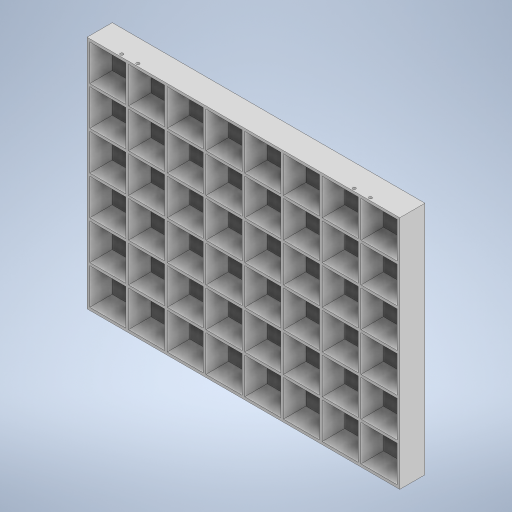
# Autodesk Inventor part: RatPelletBox_v05
Saved by Autodesk Inventor 2024 (Build 280153000, 153)
## iProperties
Created: 2025-06-19
Part Number: RatPelletBox_v05
Material: Generic
Document SubType Name: Modeling
Designer: Akramilab
Density: 1 g/cm^3
Appearance: Default
Author: Akramilab
Autodesk Inventor part; units mm, degrees
ref_plane "YZ Plane" through (0, 0, 0) normal (1, 0, 0) x (0, 1, 0)
ref_plane "XZ Plane" through (0, 0, 0) normal (0, 1, 0) x (-1, 0, 0)
ref_plane "XY Plane" through (0, 0, 0) normal (0, 0, 1) x (1, 0, 0)
sketch "Sketch1" plane through (0, 0, 0) normal (0, 0, 1) x (1, 0, 0)
  line L0 (-173.5, -130.5) -> (173.5, -130.5)
  line L1 (173.5, -130.5) -> (173.5, 130.5)
  line L2 (173.5, 130.5) -> (-173.5, 130.5)
  line L3 (-173.5, 130.5) -> (-173.5, -130.5)
  line L4 (-173.5, -130.5) -> (173.5, 130.5) construction
  line L5 (173.5, -130.5) -> (-173.5, 130.5) construction
  point P0 (0, 0)
  dimension "d0" = 347
  dimension "d1" = 261
  constraints: 12 end point, 2 midpoint, 2 parallel, 1 horizontal, 1 perpendicular
  measures "d0" distance of L1.end L2.end
  measures "d1" distance of L0.end L1.end
extrude "Extrusion1" add sketch "Sketch1" along normal blind 28
sketch "Sketch2" plane through (0, 0, 28) normal (0, 0, 1) x (1, 0, 0)
  line L0 (-170.5, 127.5) -> (-130.5, 127.5)
  line L1 (-130.5, 127.5) -> (-130.5, 87.5)
  line L2 (-130.5, 87.5) -> (-170.5, 87.5)
  line L3 (-170.5, 87.5) -> (-170.5, 127.5)
  line L4 (-170.5, 127.5) -> (-130.5, 87.5) construction
  line L5 (-130.5, 127.5) -> (-170.5, 87.5) construction
  line L6 (173.5, 130.5) -> (-173.5, 130.5) projected
  line L7 (-173.5, 130.5) -> (-173.5, -130.5) projected
  line L8 (-127.5, 127.5) -> (-87.5, 127.5)
  line L9 (-87.5, 127.5) -> (-87.5, 87.5)
  line L10 (-87.5, 87.5) -> (-127.5, 87.5)
  line L11 (-127.5, 87.5) -> (-127.5, 127.5)
  line L12 (-127.5, 127.5) -> (-87.5, 87.5) construction
  line L13 (-87.5, 127.5) -> (-127.5, 87.5) construction
  line L14 (-84.5, 127.5) -> (-44.5, 127.5)
  line L15 (-44.5, 127.5) -> (-44.5, 87.5)
  line L16 (-44.5, 87.5) -> (-84.5, 87.5)
  line L17 (-84.5, 87.5) -> (-84.5, 127.5)
  line L18 (-84.5, 127.5) -> (-44.5, 87.5) construction
  line L19 (-44.5, 127.5) -> (-84.5, 87.5) construction
  line L20 (-41.5, 127.5) -> (-1.5, 127.5)
  line L21 (-1.5, 127.5) -> (-1.5, 87.5)
  line L22 (-1.5, 87.5) -> (-41.5, 87.5)
  line L23 (-41.5, 87.5) -> (-41.5, 127.5)
  line L24 (-41.5, 127.5) -> (-1.5, 87.5) construction
  line L25 (-1.5, 127.5) -> (-41.5, 87.5) construction
  line L26 (1.5, 127.5) -> (41.5, 127.5)
  line L27 (41.5, 127.5) -> (41.5, 87.5)
  line L28 (41.5, 87.5) -> (1.5, 87.5)
  line L29 (1.5, 87.5) -> (1.5, 127.5)
  line L30 (1.5, 127.5) -> (41.5, 87.5) construction
  line L31 (41.5, 127.5) -> (1.5, 87.5) construction
  line L32 (-170.5, 84.5) -> (-130.5, 84.5)
  line L33 (-130.5, 84.5) -> (-130.5, 44.5)
  line L34 (-130.5, 44.5) -> (-170.5, 44.5)
  line L35 (-170.5, 44.5) -> (-170.5, 84.5)
  line L36 (-170.5, 84.5) -> (-130.5, 44.5) construction
  line L37 (-130.5, 84.5) -> (-170.5, 44.5) construction
  line L38 (-127.5, 84.5) -> (-87.5, 84.5)
  line L39 (-87.5, 84.5) -> (-87.5, 44.5)
  line L40 (-87.5, 44.5) -> (-127.5, 44.5)
  line L41 (-127.5, 44.5) -> (-127.5, 84.5)
  line L42 (-127.5, 84.5) -> (-87.5, 44.5) construction
  line L43 (-87.5, 84.5) -> (-127.5, 44.5) construction
  line L44 (-84.5, 84.5) -> (-44.5, 84.5)
  line L45 (-44.5, 84.5) -> (-44.5, 44.5)
  line L46 (-44.5, 44.5) -> (-84.5, 44.5)
  line L47 (-84.5, 44.5) -> (-84.5, 84.5)
  line L48 (-84.5, 84.5) -> (-44.5, 44.5) construction
  line L49 (-44.5, 84.5) -> (-84.5, 44.5) construction
  line L50 (-41.5, 84.5) -> (-1.5, 84.5)
  line L51 (-1.5, 84.5) -> (-1.5, 44.5)
  line L52 (-1.5, 44.5) -> (-41.5, 44.5)
  line L53 (-41.5, 44.5) -> (-41.5, 84.5)
  line L54 (-41.5, 84.5) -> (-1.5, 44.5) construction
  line L55 (-1.5, 84.5) -> (-41.5, 44.5) construction
  line L56 (1.5, 84.5) -> (41.5, 84.5)
  line L57 (41.5, 84.5) -> (41.5, 44.5)
  line L58 (41.5, 44.5) -> (1.5, 44.5)
  line L59 (1.5, 44.5) -> (1.5, 84.5)
  line L60 (1.5, 84.5) -> (41.5, 44.5) construction
  line L61 (41.5, 84.5) -> (1.5, 44.5) construction
  line L62 (-170.5, 41.5) -> (-130.5, 41.5)
  line L63 (-130.5, 41.5) -> (-130.5, 1.5)
  line L64 (-130.5, 1.5) -> (-170.5, 1.5)
  line L65 (-170.5, 1.5) -> (-170.5, 41.5)
  line L66 (-170.5, 41.5) -> (-130.5, 1.5) construction
  line L67 (-130.5, 41.5) -> (-170.5, 1.5) construction
  line L68 (-127.5, 41.5) -> (-87.5, 41.5)
  line L69 (-87.5, 41.5) -> (-87.5, 1.5)
  line L70 (-87.5, 1.5) -> (-127.5, 1.5)
  line L71 (-127.5, 1.5) -> (-127.5, 41.5)
  line L72 (-127.5, 41.5) -> (-87.5, 1.5) construction
  line L73 (-87.5, 41.5) -> (-127.5, 1.5) construction
  line L74 (-84.5, 41.5) -> (-44.5, 41.5)
  line L75 (-44.5, 41.5) -> (-44.5, 1.5)
  line L76 (-44.5, 1.5) -> (-84.5, 1.5)
  line L77 (-84.5, 1.5) -> (-84.5, 41.5)
  line L78 (-84.5, 41.5) -> (-44.5, 1.5) construction
  line L79 (-44.5, 41.5) -> (-84.5, 1.5) construction
  line L80 (-41.5, 41.5) -> (-1.5, 41.5)
  line L81 (-1.5, 41.5) -> (-1.5, 1.5)
  line L82 (-1.5, 1.5) -> (-41.5, 1.5)
  line L83 (-41.5, 1.5) -> (-41.5, 41.5)
  line L84 (-41.5, 41.5) -> (-1.5, 1.5) construction
  line L85 (-1.5, 41.5) -> (-41.5, 1.5) construction
  line L86 (1.5, 41.5) -> (41.5, 41.5)
  line L87 (41.5, 41.5) -> (41.5, 1.5)
  line L88 (41.5, 1.5) -> (1.5, 1.5)
  line L89 (1.5, 1.5) -> (1.5, 41.5)
  line L90 (1.5, 41.5) -> (41.5, 1.5) construction
  line L91 (41.5, 41.5) -> (1.5, 1.5) construction
  line L92 (-170.5, -1.5) -> (-130.5, -1.5)
  line L93 (-130.5, -1.5) -> (-130.5, -41.5)
  line L94 (-130.5, -41.5) -> (-170.5, -41.5)
  line L95 (-170.5, -41.5) -> (-170.5, -1.5)
  line L96 (-170.5, -1.5) -> (-130.5, -41.5) construction
  line L97 (-130.5, -1.5) -> (-170.5, -41.5) construction
  line L98 (-127.5, -1.5) -> (-87.5, -1.5)
  line L99 (-87.5, -1.5) -> (-87.5, -41.5)
  line L100 (-87.5, -41.5) -> (-127.5, -41.5)
  line L101 (-127.5, -41.5) -> (-127.5, -1.5)
  line L102 (-127.5, -1.5) -> (-87.5, -41.5) construction
  line L103 (-87.5, -1.5) -> (-127.5, -41.5) construction
  line L104 (-84.5, -1.5) -> (-44.5, -1.5)
  line L105 (-44.5, -1.5) -> (-44.5, -41.5)
  line L106 (-44.5, -41.5) -> (-84.5, -41.5)
  line L107 (-84.5, -41.5) -> (-84.5, -1.5)
  line L108 (-84.5, -1.5) -> (-44.5, -41.5) construction
  line L109 (-44.5, -1.5) -> (-84.5, -41.5) construction
  line L110 (-41.5, -1.5) -> (-1.5, -1.5)
  line L111 (-1.5, -1.5) -> (-1.5, -41.5)
  line L112 (-1.5, -41.5) -> (-41.5, -41.5)
  line L113 (-41.5, -41.5) -> (-41.5, -1.5)
  line L114 (-41.5, -1.5) -> (-1.5, -41.5) construction
  line L115 (-1.5, -1.5) -> (-41.5, -41.5) construction
  line L116 (1.5, -1.5) -> (41.5, -1.5)
  line L117 (41.5, -1.5) -> (41.5, -41.5)
  line L118 (41.5, -41.5) -> (1.5, -41.5)
  line L119 (1.5, -41.5) -> (1.5, -1.5)
  line L120 (1.5, -1.5) -> (41.5, -41.5) construction
  line L121 (41.5, -1.5) -> (1.5, -41.5) construction
  line L122 (44.5, 127.5) -> (84.5, 127.5)
  line L123 (84.5, 127.5) -> (84.5, 87.5)
  line L124 (84.5, 87.5) -> (44.5, 87.5)
  line L125 (44.5, 87.5) -> (44.5, 127.5)
  line L126 (44.5, 127.5) -> (84.5, 87.5) construction
  line L127 (84.5, 127.5) -> (44.5, 87.5) construction
  line L128 (44.5, 84.5) -> (84.5, 84.5)
  line L129 (84.5, 84.5) -> (84.5, 44.5)
  line L130 (84.5, 44.5) -> (44.5, 44.5)
  line L131 (44.5, 44.5) -> (44.5, 84.5)
  line L132 (44.5, 84.5) -> (84.5, 44.5) construction
  line L133 (84.5, 84.5) -> (44.5, 44.5) construction
  line L134 (44.5, 41.5) -> (84.5, 41.5)
  line L135 (84.5, 41.5) -> (84.5, 1.5)
  line L136 (84.5, 1.5) -> (44.5, 1.5)
  line L137 (44.5, 1.5) -> (44.5, 41.5)
  line L138 (44.5, 41.5) -> (84.5, 1.5) construction
  line L139 (84.5, 41.5) -> (44.5, 1.5) construction
  line L140 (44.5, -1.5) -> (84.5, -1.5)
  line L141 (84.5, -1.5) -> (84.5, -41.5)
  line L142 (84.5, -41.5) -> (44.5, -41.5)
  line L143 (44.5, -41.5) -> (44.5, -1.5)
  line L144 (44.5, -1.5) -> (84.5, -41.5) construction
  line L145 (84.5, -1.5) -> (44.5, -41.5) construction
  line L146 (87.5, 127.5) -> (127.5, 127.5)
  line L147 (127.5, 127.5) -> (127.5, 87.5)
  line L148 (127.5, 87.5) -> (87.5, 87.5)
  line L149 (87.5, 87.5) -> (87.5, 127.5)
  line L150 (87.5, 127.5) -> (127.5, 87.5) construction
  line L151 (127.5, 127.5) -> (87.5, 87.5) construction
  line L152 (87.5, 84.5) -> (127.5, 84.5)
  line L153 (127.5, 84.5) -> (127.5, 44.5)
  line L154 (127.5, 44.5) -> (87.5, 44.5)
  line L155 (87.5, 44.5) -> (87.5, 84.5)
  line L156 (87.5, 84.5) -> (127.5, 44.5) construction
  line L157 (127.5, 84.5) -> (87.5, 44.5) construction
  line L158 (87.5, 41.5) -> (127.5, 41.5)
  line L159 (127.5, 41.5) -> (127.5, 1.5)
  line L160 (127.5, 1.5) -> (87.5, 1.5)
  line L161 (87.5, 1.5) -> (87.5, 41.5)
  line L162 (87.5, 41.5) -> (127.5, 1.5) construction
  line L163 (127.5, 41.5) -> (87.5, 1.5) construction
  line L164 (87.5, -1.5) -> (127.5, -1.5)
  line L165 (127.5, -1.5) -> (127.5, -41.5)
  line L166 (127.5, -41.5) -> (87.5, -41.5)
  line L167 (87.5, -41.5) -> (87.5, -1.5)
  line L168 (87.5, -1.5) -> (127.5, -41.5) construction
  line L169 (127.5, -1.5) -> (87.5, -41.5) construction
  line L170 (130.5, 127.5) -> (170.5, 127.5)
  line L171 (170.5, 127.5) -> (170.5, 87.5)
  line L172 (170.5, 87.5) -> (130.5, 87.5)
  line L173 (130.5, 87.5) -> (130.5, 127.5)
  line L174 (130.5, 127.5) -> (170.5, 87.5) construction
  line L175 (170.5, 127.5) -> (130.5, 87.5) construction
  line L176 (130.5, 84.5) -> (170.5, 84.5)
  line L177 (170.5, 84.5) -> (170.5, 44.5)
  line L178 (170.5, 44.5) -> (130.5, 44.5)
  line L179 (130.5, 44.5) -> (130.5, 84.5)
  line L180 (130.5, 84.5) -> (170.5, 44.5) construction
  line L181 (170.5, 84.5) -> (130.5, 44.5) construction
  line L182 (130.5, 41.5) -> (170.5, 41.5)
  line L183 (170.5, 41.5) -> (170.5, 1.5)
  line L184 (170.5, 1.5) -> (130.5, 1.5)
  line L185 (130.5, 1.5) -> (130.5, 41.5)
  line L186 (130.5, 41.5) -> (170.5, 1.5) construction
  line L187 (170.5, 41.5) -> (130.5, 1.5) construction
  line L188 (130.5, -1.5) -> (170.5, -1.5)
  line L189 (170.5, -1.5) -> (170.5, -41.5)
  line L190 (170.5, -41.5) -> (130.5, -41.5)
  line L191 (130.5, -41.5) -> (130.5, -1.5)
  line L192 (130.5, -1.5) -> (170.5, -41.5) construction
  line L193 (170.5, -1.5) -> (130.5, -41.5) construction
  line L194 (-170.5, -44.5) -> (-130.5, -44.5)
  line L195 (-130.5, -44.5) -> (-130.5, -84.5)
  line L196 (-130.5, -84.5) -> (-170.5, -84.5)
  line L197 (-170.5, -84.5) -> (-170.5, -44.5)
  line L198 (-170.5, -44.5) -> (-130.5, -84.5) construction
  line L199 (-130.5, -44.5) -> (-170.5, -84.5) construction
  line L200 (-127.5, -44.5) -> (-87.5, -44.5)
  line L201 (-87.5, -44.5) -> (-87.5, -84.5)
  line L202 (-87.5, -84.5) -> (-127.5, -84.5)
  line L203 (-127.5, -84.5) -> (-127.5, -44.5)
  line L204 (-127.5, -44.5) -> (-87.5, -84.5) construction
  line L205 (-87.5, -44.5) -> (-127.5, -84.5) construction
  line L206 (-84.5, -44.5) -> (-44.5, -44.5)
  line L207 (-44.5, -44.5) -> (-44.5, -84.5)
  line L208 (-44.5, -84.5) -> (-84.5, -84.5)
  line L209 (-84.5, -84.5) -> (-84.5, -44.5)
  line L210 (-84.5, -44.5) -> (-44.5, -84.5) construction
  line L211 (-44.5, -44.5) -> (-84.5, -84.5) construction
  line L212 (-41.5, -44.5) -> (-1.5, -44.5)
  line L213 (-1.5, -44.5) -> (-1.5, -84.5)
  line L214 (-1.5, -84.5) -> (-41.5, -84.5)
  line L215 (-41.5, -84.5) -> (-41.5, -44.5)
  line L216 (-41.5, -44.5) -> (-1.5, -84.5) construction
  line L217 (-1.5, -44.5) -> (-41.5, -84.5) construction
  line L218 (1.5, -44.5) -> (41.5, -44.5)
  line L219 (41.5, -44.5) -> (41.5, -84.5)
  line L220 (41.5, -84.5) -> (1.5, -84.5)
  line L221 (1.5, -84.5) -> (1.5, -44.5)
  line L222 (1.5, -44.5) -> (41.5, -84.5) construction
  line L223 (41.5, -44.5) -> (1.5, -84.5) construction
  line L224 (44.5, -44.5) -> (84.5, -44.5)
  line L225 (84.5, -44.5) -> (84.5, -84.5)
  line L226 (84.5, -84.5) -> (44.5, -84.5)
  line L227 (44.5, -84.5) -> (44.5, -44.5)
  line L228 (44.5, -44.5) -> (84.5, -84.5) construction
  line L229 (84.5, -44.5) -> (44.5, -84.5) construction
  line L230 (87.5, -44.5) -> (127.5, -44.5)
  line L231 (127.5, -44.5) -> (127.5, -84.5)
  line L232 (127.5, -84.5) -> (87.5, -84.5)
  line L233 (87.5, -84.5) -> (87.5, -44.5)
  line L234 (87.5, -44.5) -> (127.5, -84.5) construction
  line L235 (127.5, -44.5) -> (87.5, -84.5) construction
  line L236 (130.5, -44.5) -> (170.5, -44.5)
  line L237 (170.5, -44.5) -> (170.5, -84.5)
  line L238 (170.5, -84.5) -> (130.5, -84.5)
  line L239 (130.5, -84.5) -> (130.5, -44.5)
  line L240 (130.5, -44.5) -> (170.5, -84.5) construction
  line L241 (170.5, -44.5) -> (130.5, -84.5) construction
  line L242 (-170.5, -87.5) -> (-130.5, -87.5)
  line L243 (-130.5, -87.5) -> (-130.5, -127.5)
  line L244 (-130.5, -127.5) -> (-170.5, -127.5)
  line L245 (-170.5, -127.5) -> (-170.5, -87.5)
  line L246 (-170.5, -87.5) -> (-130.5, -127.5) construction
  line L247 (-130.5, -87.5) -> (-170.5, -127.5) construction
  line L248 (-127.5, -87.5) -> (-87.5, -87.5)
  line L249 (-87.5, -87.5) -> (-87.5, -127.5)
  line L250 (-87.5, -127.5) -> (-127.5, -127.5)
  line L251 (-127.5, -127.5) -> (-127.5, -87.5)
  line L252 (-127.5, -87.5) -> (-87.5, -127.5) construction
  line L253 (-87.5, -87.5) -> (-127.5, -127.5) construction
  line L254 (-84.5, -87.5) -> (-44.5, -87.5)
  line L255 (-44.5, -87.5) -> (-44.5, -127.5)
  line L256 (-44.5, -127.5) -> (-84.5, -127.5)
  line L257 (-84.5, -127.5) -> (-84.5, -87.5)
  line L258 (-84.5, -87.5) -> (-44.5, -127.5) construction
  line L259 (-44.5, -87.5) -> (-84.5, -127.5) construction
  line L260 (-41.5, -87.5) -> (-1.5, -87.5)
  line L261 (-1.5, -87.5) -> (-1.5, -127.5)
  line L262 (-1.5, -127.5) -> (-41.5, -127.5)
  line L263 (-41.5, -127.5) -> (-41.5, -87.5)
  line L264 (-41.5, -87.5) -> (-1.5, -127.5) construction
  line L265 (-1.5, -87.5) -> (-41.5, -127.5) construction
  line L266 (1.5, -87.5) -> (41.5, -87.5)
  line L267 (41.5, -87.5) -> (41.5, -127.5)
  line L268 (41.5, -127.5) -> (1.5, -127.5)
  line L269 (1.5, -127.5) -> (1.5, -87.5)
  line L270 (1.5, -87.5) -> (41.5, -127.5) construction
  line L271 (41.5, -87.5) -> (1.5, -127.5) construction
  line L272 (44.5, -87.5) -> (84.5, -87.5)
  line L273 (84.5, -87.5) -> (84.5, -127.5)
  line L274 (84.5, -127.5) -> (44.5, -127.5)
  line L275 (44.5, -127.5) -> (44.5, -87.5)
  line L276 (44.5, -87.5) -> (84.5, -127.5) construction
  line L277 (84.5, -87.5) -> (44.5, -127.5) construction
  line L278 (87.5, -87.5) -> (127.5, -87.5)
  line L279 (127.5, -87.5) -> (127.5, -127.5)
  line L280 (127.5, -127.5) -> (87.5, -127.5)
  line L281 (87.5, -127.5) -> (87.5, -87.5)
  line L282 (87.5, -87.5) -> (127.5, -127.5) construction
  line L283 (127.5, -87.5) -> (87.5, -127.5) construction
  line L284 (130.5, -87.5) -> (170.5, -87.5)
  line L285 (170.5, -87.5) -> (170.5, -127.5)
  line L286 (170.5, -127.5) -> (130.5, -127.5)
  line L287 (130.5, -127.5) -> (130.5, -87.5)
  line L288 (130.5, -87.5) -> (170.5, -127.5) construction
  line L289 (170.5, -87.5) -> (130.5, -127.5) construction
  point P0 (0, 0)
  point P1 (-150.5, 107.5)
  point P2 (-107.5, 107.5)
  point P3 (-64.5, 107.5)
  point P4 (-21.5, 107.5)
  point P5 (21.5, 107.5)
  point P6 (-150.5, 64.5)
  point P7 (-107.5, 64.5)
  point P8 (-64.5, 64.5)
  point P9 (-21.5, 64.5)
  point P10 (21.5, 64.5)
  point P11 (-150.5, 21.5)
  point P12 (-107.5, 21.5)
  point P13 (-64.5, 21.5)
  point P14 (-21.5, 21.5)
  point P15 (21.5, 21.5)
  point P16 (-150.5, -21.5)
  point P17 (-107.5, -21.5)
  point P18 (-64.5, -21.5)
  point P19 (-21.5, -21.5)
  point P20 (21.5, -21.5)
  point P21 (64.5, 107.5)
  point P22 (64.5, 64.5)
  point P23 (64.5, 21.5)
  point P24 (64.5, -21.5)
  point P25 (107.5, 107.5)
  point P26 (107.5, 64.5)
  point P27 (107.5, 21.5)
  point P28 (107.5, -21.5)
  point P29 (150.5, 107.5)
  point P30 (150.5, 64.5)
  point P31 (150.5, 21.5)
  point P32 (150.5, -21.5)
  point P33 (-150.5, -64.5)
  point P34 (-107.5, -64.5)
  point P35 (-64.5, -64.5)
  point P36 (-21.5, -64.5)
  point P37 (21.5, -64.5)
  point P38 (64.5, -64.5)
  point P39 (107.5, -64.5)
  point P40 (150.5, -64.5)
  point P41 (-150.5, -107.5)
  point P42 (-107.5, -107.5)
  point P43 (-64.5, -107.5)
  point P44 (-21.5, -107.5)
  point P45 (21.5, -107.5)
  point P46 (64.5, -107.5)
  point P47 (107.5, -107.5)
  point P48 (150.5, -107.5)
  dimension "d4" = 40
  dimension "d5" = 3
  dimension "d6" = 3
  dimension "d7" = 40
  dimension "d10" = 43
  dimension "d13" = 43
  constraints: 576 end point, 2 collinear, 2 horizontal, 2 midpoint, 2 parallel, 1 perpendicular, 1 vertical, 515 other
  measures "d4" distance of L0.start L0.end
  measures "d5" distance between parallel lines of L6 L0
  measures "d6" distance between parallel lines of L7 L3
  measures "d7" distance of L0.end L1.end
  measures "d10" distance of L0.start L8.start
  measures "d13" distance of L0.start L32.start
extrude "Extrusion2" cut sketch "Sketch2" against normal blind 25
sketch "Sketch3" plane through (-173.5, 130.5, 0) normal (0, 1, 0) x (1, 0, 0)
  line L0 (46, -28) -> (46, -3) construction
  line L1 (43, -28) -> (43, -3) construction
  line L2 (43, -28) -> (43, -3) projected
  line L3 (43, -25) -> (46, -25) construction
  line L4 (46, -28) -> (46, -3) projected
  line L5 (347, -28) -> (0, -28) projected
  circle A0 centre (53.5, -25) radius 1.65
  circle A1 centre (35.5, -25) radius 1.65
  line L6 (172, -28) -> (172, -3) construction
  line L7 (175, -28) -> (175, -3) construction
  circle A2 centre (311.5, -25) radius 1.65
  circle A3 centre (293.5, -25) radius 1.65
  line L8 (347, 0) -> (347, -28) projected
  point P0 (173.5, 0)
  point P1 (44.5, -25)
  dimension "d20" = 3
  dimension "d21" = 3.3
  dimension "d22" = 9
  dimension "d23" = 3.3
  dimension "d24" = 9
  dimension "d25" = 3.3
  dimension "d31" = 3.3
  dimension "d35" = 18
  dimension "d36" = 35.5
  constraints: 4 centre point, 4 point on line, 2 end point, 1 midpoint, 1 perpendicular
  measures "d20" distance from line of L5 point (44.5, -25)
  measures "d21" diameter of A0
  measures "d22" distance of A0.centre point (44.5, -25)
  measures "d23" diameter of A1
  measures "d24" distance of A1.centre point (44.5, -25)
  measures "d25" diameter of A2
  measures "d31" diameter of A3
  measures "d35" distance of A2.centre A3.centre
  measures "d36" distance from line of A2.centre L8
extrude "Extrusion3" cut sketch "Sketch3" against normal blind 10
equation "\"d0\" = box_length"
equation "\"d1\" = box_width"
equation "\"d2\" = hole_height + wall"
equation "\"d4\" = hole"
equation "\"d5\" = wall"
equation "\"d6\" = wall"
equation "\"d7\" = hole"
equation "\"d10\" = hole + wall"
equation "\"d13\" = hole + wall"
equation "\"d16\" = hole_height"
equation "\"d23\" = d21"
equation "\"d24\" = d22"
equation "\"d25\" = d21"
equation "\"d31\" = d25"
equation "\"hole\" = 40"
equation "\"wall\" = 3"
equation "\"hole_height\" = 25"
equation "\"box_length\" = 347"
equation "\"box_width\" = 261"
body "Solid1"
